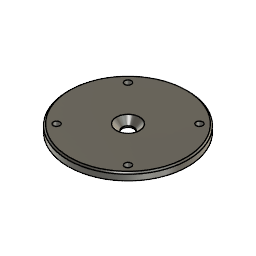
WeatherLox-Wind-Adapter (Autodesk Fusion 360 design; units mm, degrees)
Autodesk Fusion 360 part; units mm, degrees
sketch "Skizze1" plane through (0, 0, 0) normal (0, 0, 1) x (1, 0, 0)
  circle A0 centre (0, 0) radius 41
  circle A1 centre (24.5, 24.5) radius 2.25
  circle A2 centre (24.5, -24.5) radius 2.25
  circle A3 centre (-24.5, -24.5) radius 2.25
  circle A4 centre (-24.5, 24.5) radius 2.25
  dimension "d1" = 82
  dimension "d4" = 49
  dimension "d5" = 49
  dimension "d6" = 4.5
  dimension "d7" = 4.5
  dimension "d8" = 4.5
  dimension "d9" = 4.5
  constraint coincident A0.centre origin
  measures "d1" diameter of A0
  measures "d4" distance of A1.centre A4.centre
  measures "d5" distance of A3.centre A4.centre
  measures "d6" diameter of A1
  measures "d7" diameter of A2
  measures "d8" diameter of A3
  measures "d9" diameter of A4
extrude "Extrusion1" add sketch "Skizze1" along normal blind 5
chamfer "Fase1" distance 1 angle 45 1 edges at (-38.2254, -14.8262, 5)
sketch "Skizze2" plane through (0, 0, 5) normal (0, 0, 1) x (-1, 0, 0)
  circle A0 centre (-24.5, -24.5) radius 2.25
  circle A1 centre (24.5, 24.5) radius 2.25
  circle A2 centre (-24.5, 24.5) radius 2.25
  circle A3 centre (24.5, -24.5) radius 2.25
  circle A4 centre (0, 0) radius 40
  constraint coincident A4.centre origin
hole "Bohrung1" at (0, 0, 5) direction (0, 0, -1) diameter 8 depth 5 tip angle 118 countersink diameter 16 countersink angle 90
